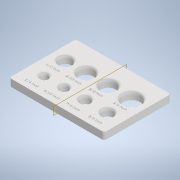
# Autodesk Inventor part: inchHexSocketSetOf8
Saved by Autodesk Inventor 2020.3 (Build 243373000, 373)
## iProperties
Created: 2020-03-13
Part Number: inchHexSocketSetOf8
Material: Generic
Document SubType Name: Modeling
Designer: robst
Density: 1 g/cm^3
Appearance: Default
Author: robst
Autodesk Inventor part; units mm, degrees
(part 1 of 2)
ref_plane "XZ Plane" through (0, 0, 0) normal (0, 1, 0) x (-1, 0, 0)
ref_plane "XY Plane" through (0, 0, 0) normal (0, 0, 1) x (1, 0, 0)
sketch "Sketch1" plane through (0, 0, 0) normal (0, 1, 0) x (-1, 0, 0)
  line L0 (63.5, 44.45) -> (-63.5, 44.45)
  line L1 (-63.5, 44.45) -> (-63.5, -44.45)
  line L2 (-63.5, -44.45) -> (63.5, -44.45)
  line L3 (63.5, -44.45) -> (63.5, 44.45)
  line L4 (63.5, 44.45) -> (-63.5, -44.45) construction
  line L5 (-63.5, 44.45) -> (63.5, -44.45) construction
  point P0 (0, 0)
  dimension "d3" = 88.9
  dimension "d13" = 127
  constraints: 12 end point, 2 midpoint, 2 parallel, 1 horizontal, 1 perpendicular
  measures "d3" distance of L2.end L0.start
  measures "d13" distance of L1.end L2.end
extrude "Extrusion1" add sketch "Sketch1" against normal blind 9.525
sketch "Sketch4" plane through (0, 0, 0) normal (0, 1, 0) x (1, 0, 0)
  line L0 (-63.5, -44.45) -> (-63.5, 44.45) construction
  line L1 (-63.5, -19.05) -> (63.5, -19.05) construction
  line L2 (63.5, 44.45) -> (63.5, -44.45) construction
  line L3 (-63.5, -44.45) -> (63.5, -44.45) projected
  circle A0 centre (-42.0827, -19.05) radius 4.699
  circle A1 centre (-15.4584, -19.05) radius 5.207
  circle A2 centre (12.6898, -19.05) radius 6.223
  circle A3 centre (42.7431, -19.05) radius 7.112
  line L4 (-63.5, 12.7) -> (63.5, 12.7) construction
  circle A4 centre (-45.6692, 12.7) radius 8.128
  circle A5 centre (-17.8054, 12.7) radius 10.033
  circle A6 centre (11.8364, 12.7) radius 9.906
  circle A7 centre (43.0657, 12.7) radius 11.6205
  point P0 (0, 0)
  dimension "d16" = 25.4
  dimension "hex1_4inchHole" = 9.398
  dimension "gap0" = 16.7183
  dimension "hex5_16inchHole" = 10.414
  dimension "gap1" = 26.6243
  dimension "hex3_8inchHole" = 12.446
  dimension "gap2" = 28.1483
  dimension "gap3" = 30.0533
  dimension "hex7_16inchHole" = 14.224
  dimension "frontToBackRowGap" = 31.75
  dimension "gap5" = 9.7028
  dimension "hex1_2inchHole" = 16.256
  dimension "hex9_16inchHole" = 20.066
  dimension "gap6" = 27.8638
  dimension "hex5_8inchHole" = 19.812
  dimension "gap7" = 29.6418
  dimension "hex3_4inchHole" = 23.241
  dimension "gap8" = 31.2293
  dimension "d37" = 8.8138
  dimension "d57" = 13.6449
  constraints: 12 point on line, 8 centre point, 4 end point, 1 horizontal, 1 perpendicular
  measures "d16" distance between parallel lines of L1 L3
  measures "hex1_4inchHole" diameter of A0
  measures "gap0" distance edge to line of A0 L0
  measures "hex5_16inchHole" diameter of A1
  measures "gap1" distance of A1.centre A0.centre
  measures "hex3_8inchHole" diameter of A2
  measures "gap2" distance of A2.centre A1.centre
  measures "gap3" distance of A3.centre A2.centre
  measures "hex7_16inchHole" diameter of A3
  measures "frontToBackRowGap" distance between parallel lines of L4 L1
  measures "gap5" distance edge to line of A4 L0
  measures "hex1_2inchHole" diameter of A4
  measures "hex9_16inchHole" diameter of A5
  measures "gap6" distance of A5.centre A4.centre
  measures "hex5_8inchHole" diameter of A6
  measures "gap7" distance of A6.centre A5.centre
  measures "hex3_4inchHole" diameter of A7
  measures "gap8" distance of A7.centre A6.centre
  measures "d37" distance edge to line of A7 L2
  measures "d57" distance edge to line of A3 L2
extrude "Extrusion3" cut sketch "Sketch4" against normal through all
sketch "Sketch7" plane through (0, 0, 0) normal (0, 1, 0) x (1, 0, 0)
  circle A0 centre (-42.0827, -19.05) radius 4.699 construction
  line L0 (63.5, -44.45) -> (-63.5, -44.45) construction
  line L1 (-46.7817, -35.6779) -> (-37.3837, -35.6779) construction
  line L2 (-20.6654, -35.6779) -> (-10.2514, -35.6779) construction
  line L3 (6.4668, -35.6779) -> (18.9128, -35.6779) construction
  line L4 (35.6311, -35.6779) -> (49.8551, -35.6779) construction
  line L5 (-53.7972, -3.81) -> (-37.5412, -3.81) construction
  line L6 (-27.8384, -3.9984) -> (-7.7724, -3.9984) construction
  line L7 (1.9304, -3.8276) -> (21.7424, -3.8276) construction
  line L8 (31.4452, -3.6244) -> (56.0832, -3.6244) construction
  line L9 (-20.6654, -35.6779) -> (-20.6654, -19.05) construction
  circle A1 centre (-15.4584, -19.05) radius 5.207 construction
  line L10 (-10.2514, -35.6779) -> (-10.2514, -19.05) construction
  line L11 (-46.7817, -19.05) -> (-46.7817, -35.6779) construction
  line L12 (-37.3837, -35.6779) -> (-37.3837, -19.05) construction
  line L13 (6.4668, -35.6779) -> (6.4668, -19.05) construction
  circle A2 centre (12.6898, -19.05) radius 6.223 construction
  line L14 (18.9128, -35.6779) -> (18.9128, -19.05) construction
  line L15 (49.8551, -35.6779) -> (49.8551, -19.05) construction
  circle A3 centre (42.7431, -19.05) radius 7.112 construction
  line L16 (35.6311, -35.6779) -> (35.6311, -19.05) construction
  circle A4 centre (-45.6692, 12.7) radius 8.128 construction
  line L17 (-53.7972, 12.7) -> (-53.7972, -3.81) construction
  line L18 (-37.5412, 12.7) -> (-37.5412, -3.81) construction
  circle A5 centre (-17.8054, 12.7) radius 10.033 construction
  line L19 (-27.8384, 12.7) -> (-27.8384, -3.9984) construction
  line L20 (-7.7724, 12.7) -> (-7.7724, -3.9984) construction
  circle A6 centre (11.8364, 12.7) radius 9.906 construction
  line L21 (1.9304, 12.7) -> (1.9304, -3.8276) construction
  line L22 (21.7424, 12.7) -> (21.7424, -3.8276) construction
  circle A7 centre (43.0657, 12.7) radius 11.6205 construction
  line L23 (31.4452, 12.7) -> (31.4452, -3.6244) construction
  line L24 (56.0832, 12.702) -> (56.0832, -3.6244) construction
  line L25 (-52.169, -5.334) -> (-54.1821, -5.334)
  line L26 (-54.1821, -5.334) -> (-54.1821, -4.8029)
  line L27 (-54.1821, -4.8029) -> (-53.5399, -4.8029)
  line L28 (-53.5399, -4.8029) -> (-53.5399, -3.19)
  line L29 (-53.5399, -3.19) -> (-54.1821, -3.19)
  line L30 (-54.1821, -3.19) -> (-54.1821, -2.6936)
  spline S0 degree 2 poles (-54.1821, -2.6936) (-54.0413, -2.6936) (-53.7622, -2.6565) (-53.6782, -2.617) knots 0 0 0 1 2 2 2
  spline S1 degree 2 poles (-53.6782, -2.617) (-53.5819, -2.5676) (-53.4732, -2.4021) (-53.4633, -2.2786) knots 0 0 0 1 2 2 2
  line L31 (-53.4633, -2.2786) -> (-52.7964, -2.2786)
  line L32 (-52.7964, -2.2786) -> (-52.7964, -4.8029)
  line L33 (-52.7964, -4.8029) -> (-52.169, -4.8029)
  line L34 (-52.169, -4.8029) -> (-52.169, -5.334)
  line L35 (-49.8695, -2.1501) -> (-51.0822, -5.996)
  line L36 (-51.0822, -5.996) -> (-51.6701, -5.996)
  line L37 (-51.6701, -5.996) -> (-50.4598, -2.1501)
  line L38 (-50.4598, -2.1501) -> (-49.8695, -2.1501)
  line L39 (-46.945, -5.334) -> (-49.1853, -5.334)
  line L40 (-49.1853, -5.334) -> (-49.1853, -4.8375)
  spline S2 degree 2 poles (-49.1853, -4.8375) (-48.9012, -4.6103) (-48.4467, -4.2101) (-48.2763, -4.0298) knots 0 0 0 1 2 2 2
  spline S3 degree 2 poles (-48.2763, -4.0298) (-48.0515, -3.7952) (-47.8515, -3.437) (-47.8515, -3.2493) knots 0 0 0 1 2 2 2
  spline S4 degree 2 poles (-47.8515, -3.2493) (-47.8515, -3.0369) (-48.1059, -2.8096) (-48.3331, -2.8096) knots 0 0 0 1 2 2 2
  spline S5 degree 2 poles (-48.3331, -2.8096) (-48.4492, -2.8096) (-48.6567, -2.8665) (-48.7629, -2.9109) knots 0 0 0 1 2 2 2
  spline S6 degree 2 poles (-48.7629, -2.9109) (-48.8666, -2.9578) (-49.0148, -3.0566) (-49.0519, -3.0813) knots 0 0 0 1 2 2 2
  line L41 (-49.0519, -3.0813) -> (-49.1112, -3.0813)
  line L42 (-49.1112, -3.0813) -> (-49.1112, -2.4169)
  spline S7 degree 2 poles (-49.1112, -2.4169) (-48.9827, -2.3552) (-48.4344, -2.2267) (-48.18, -2.2267) knots 0 0 0 1 2 2 2
  spline S8 degree 2 poles (-48.18, -2.2267) (-47.6366, -2.2267) (-47.0783, -2.7108) (-47.0783, -3.148) knots 0 0 0 1 2 2 2
  spline S9 degree 2 poles (-47.0783, -3.148) (-47.0783, -3.4173) (-47.3328, -3.936) (-47.6267, -4.2324) knots 0 0 0 1 2 2 2
  spline S10 degree 2 poles (-47.6267, -4.2324) (-47.8119, -4.4152) (-48.1602, -4.6992) (-48.2368, -4.7585) knots 0 0 0 1 2 2 2
  line L43 (-48.2368, -4.7585) -> (-46.945, -4.7585)
  line L44 (-46.945, -4.7585) -> (-46.945, -5.334)
  line L45 (-44.6059, -5.334) -> (-45.3222, -5.334)
  line L46 (-45.3222, -5.334) -> (-45.3222, -3.0344)
  line L47 (-45.3222, -3.0344) -> (-44.6059, -3.0344)
  line L48 (-44.6059, -3.0344) -> (-44.6059, -5.334)
  line L49 (-44.5836, -2.7059) -> (-45.3419, -2.7059)
  line L50 (-45.3419, -2.7059) -> (-45.3419, -2.1477)
  line L51 (-45.3419, -2.1477) -> (-44.5836, -2.1477)
  line L52 (-44.5836, -2.1477) -> (-44.5836, -2.7059)
  line L53 (-41.9061, -5.334) -> (-42.6274, -5.334)
  line L54 (-42.6274, -5.334) -> (-42.6274, -4.1953)
  spline S11 degree 2 poles (-42.6274, -4.1953) (-42.6274, -4.0545) (-42.6496, -3.7779) (-42.6792, -3.7137) knots 0 0 0 1 2 2 2
  spline S12 degree 2 poles (-42.6792, -3.7137) (-42.7163, -3.6346) (-42.8546, -3.5679) (-42.9732, -3.5679) knots 0 0 0 1 2 2 2
  spline S13 degree 2 poles (-42.9732, -3.5679) (-43.0596, -3.5679) (-43.2399, -3.6346) (-43.3412, -3.7063) knots 0 0 0 1 2 2 2
  line L55 (-43.3412, -3.7063) -> (-43.3412, -5.334)
  line L56 (-43.3412, -5.334) -> (-44.0575, -5.334)
  line L57 (-44.0575, -5.334) -> (-44.0575, -3.0344)
  line L58 (-44.0575, -3.0344) -> (-43.3412, -3.0344)
  line L59 (-43.3412, -3.0344) -> (-43.3412, -3.2888)
  spline S14 degree 2 poles (-43.3412, -3.2888) (-43.1658, -3.1406) (-42.8324, -2.9727) (-42.6298, -2.9727) knots 0 0 0 1 2 2 2
  spline S15 degree 2 poles (-42.6298, -2.9727) (-42.2791, -2.9727) (-41.9061, -3.4173) (-41.9061, -3.8372) knots 0 0 0 1 2 2 2
  line L60 (-41.9061, -3.8372) -> (-41.9061, -5.334)
  spline S16 degree 2 poles (-40.2487, -5.3958) (-40.5328, -5.3958) (-41.0046, -5.2525) (-41.1799, -5.1043) knots 0 0 0 1 2 2 2
  spline S17 degree 2 poles (-41.1799, -5.1043) (-41.3504, -4.9536) (-41.543, -4.5016) (-41.543, -4.1953) knots 0 0 0 1 2 2 2
  spline S18 degree 2 poles (-41.543, -4.1953) (-41.543, -3.8643) (-41.3356, -3.4024) (-41.1552, -3.2542) knots 0 0 0 1 2 2 2
  spline S19 degree 2 poles (-41.1552, -3.2542) (-40.9848, -3.111) (-40.5205, -2.9727) (-40.2685, -2.9727) knots 0 0 0 1 2 2 2
  spline S20 degree 2 poles (-40.2685, -2.9727) (-40.0783, -2.9727) (-39.6979, -3.0616) (-39.5053, -3.1579) knots 0 0 0 1 2 2 2
  line L61 (-39.5053, -3.1579) -> (-39.5053, -3.7705)
  line L62 (-39.5053, -3.7705) -> (-39.5967, -3.7705)
  spline S21 degree 2 poles (-39.5967, -3.7705) (-39.6411, -3.7285) (-39.7646, -3.6297) (-39.8387, -3.5902) knots 0 0 0 1 2 2 2
  spline S22 degree 2 poles (-39.8387, -3.5902) (-39.9178, -3.5457) (-40.1129, -3.4864) (-40.2339, -3.4864) knots 0 0 0 1 2 2 2
  spline S23 degree 2 poles (-40.2339, -3.4864) (-40.5081, -3.4864) (-40.8094, -3.8693) (-40.8094, -4.1953) knots 0 0 0 1 2 2 2
  spline S24 degree 2 poles (-40.8094, -4.1953) (-40.8094, -4.5411) (-40.4883, -4.882) (-40.2216, -4.882) knots 0 0 0 1 2 2 2
  spline S25 degree 2 poles (-40.2216, -4.882) (-40.0857, -4.882) (-39.8832, -4.8202) (-39.8091, -4.7758) knots 0 0 0 1 2 2 2
  spline S26 degree 2 poles (-39.8091, -4.7758) (-39.7375, -4.7338) (-39.6337, -4.6399) (-39.5967, -4.6029) knots 0 0 0 1 2 2 2
  line L63 (-39.5967, -4.6029) -> (-39.5053, -4.6029)
  line L64 (-39.5053, -4.6029) -> (-39.5053, -5.2179)
  spline S27 degree 2 poles (-39.5053, -5.2179) (-39.567, -5.2451) (-39.7276, -5.3142) (-39.8116, -5.3365) knots 0 0 0 1 2 2 2
  spline S28 degree 2 poles (-39.8116, -5.3365) (-39.9153, -5.3661) (-40.0981, -5.3958) (-40.2487, -5.3958) knots 0 0 0 1 2 2 2
  line L65 (-37.013, -5.334) -> (-37.7343, -5.334)
  line L66 (-37.7343, -5.334) -> (-37.7343, -4.1953)
  spline S29 degree 2 poles (-37.7343, -4.1953) (-37.7343, -4.0545) (-37.7565, -3.7779) (-37.7861, -3.7137) knots 0 0 0 1 2 2 2
  spline S30 degree 2 poles (-37.7861, -3.7137) (-37.8232, -3.6346) (-37.9615, -3.5679) (-38.0801, -3.5679) knots 0 0 0 1 2 2 2
  spline S31 degree 2 poles (-38.0801, -3.5679) (-38.1665, -3.5679) (-38.3468, -3.6346) (-38.4481, -3.7063) knots 0 0 0 1 2 2 2
  line L67 (-38.4481, -3.7063) -> (-38.4481, -5.334)
  line L68 (-38.4481, -5.334) -> (-39.1644, -5.334)
  line L69 (-39.1644, -5.334) -> (-39.1644, -2.1501)
  line L70 (-39.1644, -2.1501) -> (-38.4481, -2.1501)
  line L71 (-38.4481, -2.1501) -> (-38.4481, -3.2888)
  spline S32 degree 2 poles (-38.4481, -3.2888) (-38.2727, -3.1406) (-37.9393, -2.9727) (-37.7367, -2.9727) knots 0 0 0 1 2 2 2
  spline S33 degree 2 poles (-37.7367, -2.9727) (-37.386, -2.9727) (-37.013, -3.4173) (-37.013, -3.8372) knots 0 0 0 1 2 2 2
  line L72 (-37.013, -3.8372) -> (-37.013, -5.334)
  spline S34 degree 2 poles (-25.5835, -3.828) (-25.5835, -4.2158) (-25.7638, -4.863) (-25.954, -5.0951) knots 0 0 0 1 2 2 2
  spline S35 degree 2 poles (-25.954, -5.0951) (-26.1516, -5.3298) (-26.7345, -5.5817) (-27.1594, -5.5817) knots 0 0 0 1 2 2 2
  spline S36 degree 2 poles (-27.1594, -5.5817) (-27.3026, -5.5817) (-27.6138, -5.5447) (-27.6657, -5.5299) knots 0 0 0 1 2 2 2
  line L73 (-27.6657, -5.5299) -> (-27.6657, -4.9321)
  line L74 (-27.6657, -4.9321) -> (-27.6064, -4.9321)
  spline S37 degree 2 poles (-27.6064, -4.9321) (-27.5496, -4.9618) (-27.3372, -5.026) (-27.1519, -5.026) knots 0 0 0 1 2 2 2
  spline S38 degree 2 poles (-27.1519, -5.026) (-27.0013, -5.026) (-26.7222, -4.9469) (-26.6234, -4.8605) knots 0 0 0 1 2 2 2
  spline S39 degree 2 poles (-26.6234, -4.8605) (-26.5171, -4.7691) (-26.3788, -4.4999) (-26.3541, -4.2973) knots 0 0 0 1 2 2 2
  spline S40 degree 2 poles (-26.3541, -4.2973) (-26.5171, -4.3986) (-26.7987, -4.5073) (-27.0087, -4.5073) knots 0 0 0 1 2 2 2
  spline S41 degree 2 poles (-27.0087, -4.5073) (-27.1643, -4.5073) (-27.4533, -4.4233) (-27.5718, -4.3344) knots 0 0 0 1 2 2 2
  spline S42 degree 2 poles (-27.5718, -4.3344) (-27.7299, -4.2133) (-27.9152, -3.8255) (-27.9152, -3.5193) knots 0 0 0 1 2 2 2
  spline S43 degree 2 poles (-27.9152, -3.5193) (-27.9152, -3.2797) (-27.7522, -2.8771) (-27.604, -2.7289) knots 0 0 0 1 2 2 2
  spline S44 degree 2 poles (-27.604, -2.7289) (-27.4558, -2.5807) (-27.026, -2.4127) (-26.7617, -2.4127) knots 0 0 0 1 2 2 2
  spline S45 degree 2 poles (-26.7617, -2.4127) (-26.4949, -2.4127) (-26.0824, -2.5609) (-25.9342, -2.7165) knots 0 0 0 1 2 2 2
  spline S46 degree 2 poles (-25.9342, -2.7165) (-25.7613, -2.8894) (-25.5835, -3.4378) (-25.5835, -3.828) knots 0 0 0 1 2 2 2
  spline S47 degree 2 poles (-26.3418, -3.7144) (-26.3418, -3.4649) (-26.4258, -3.1438) (-26.5023, -3.0549) knots 0 0 0 1 2 2 2
  spline S48 degree 2 poles (-26.5023, -3.0549) (-26.5542, -2.9882) (-26.6876, -2.9314) (-26.7641, -2.9314) knots 0 0 0 1 2 2 2
  spline S49 degree 2 poles (-26.7641, -2.9314) (-26.8333, -2.9314) (-26.9618, -2.9857) (-27.021, -3.0549) knots 0 0 0 1 2 2 2
  spline S50 degree 2 poles (-27.021, -3.0549) (-27.0729, -3.1142) (-27.147, -3.3439) (-27.147, -3.4797) knots 0 0 0 1 2 2 2
  spline S51 degree 2 poles (-27.147, -3.4797) (-27.147, -3.6279) (-27.0704, -3.8181) (-27.0062, -3.8749) knots 0 0 0 1 2 2 2
  spline S52 degree 2 poles (-27.0062, -3.8749) (-26.9395, -3.9318) (-26.774, -3.9762) (-26.6703, -3.9762) knots 0 0 0 1 2 2 2
  spline S53 degree 2 poles (-26.6703, -3.9762) (-26.5838, -3.9762) (-26.4035, -3.9293) (-26.3467, -3.9046) knots 0 0 0 1 2 2 2
  spline S54 degree 2 poles (-26.3467, -3.9046) (-26.3467, -3.8824) (-26.3418, -3.7984) (-26.3418, -3.7144) knots 0 0 0 1 2 2 2
  line L75 (-23.3407, -2.3386) -> (-24.5535, -6.1844)
  line L76 (-24.5535, -6.1844) -> (-25.1413, -6.1844)
  line L77 (-25.1413, -6.1844) -> (-23.931, -2.3386)
  line L78 (-23.931, -2.3386) -> (-23.3407, -2.3386)
  line L79 (-20.5521, -5.5224) -> (-22.5651, -5.5224)
  line L80 (-22.5651, -5.5224) -> (-22.5651, -4.9914)
  line L81 (-22.5651, -4.9914) -> (-21.9229, -4.9914)
  line L82 (-21.9229, -4.9914) -> (-21.9229, -3.3785)
  line L83 (-21.9229, -3.3785) -> (-22.5651, -3.3785)
  line L84 (-22.5651, -3.3785) -> (-22.5651, -2.882)
  spline S55 degree 2 poles (-22.5651, -2.882) (-22.4243, -2.882) (-22.1452, -2.8449) (-22.0612, -2.8054) knots 0 0 0 1 2 2 2
  spline S56 degree 2 poles (-22.0612, -2.8054) (-21.9649, -2.756) (-21.8562, -2.5905) (-21.8463, -2.467) knots 0 0 0 1 2 2 2
  line L85 (-21.8463, -2.467) -> (-21.1794, -2.467)
  line L86 (-21.1794, -2.467) -> (-21.1794, -4.9914)
  line L87 (-21.1794, -4.9914) -> (-20.5521, -4.9914)
  line L88 (-20.5521, -4.9914) -> (-20.5521, -5.5224)
  spline S57 degree 2 poles (-17.7634, -4.485) (-17.7634, -4.9667) (-18.3735, -5.5867) (-18.907, -5.5867) knots 0 0 0 1 2 2 2
  spline S58 degree 2 poles (-18.907, -5.5867) (-19.1738, -5.5867) (-19.5912, -5.4335) (-19.737, -5.2829) knots 0 0 0 1 2 2 2
  spline S59 degree 2 poles (-19.737, -5.2829) (-19.9099, -5.1075) (-20.0951, -4.5517) (-20.0951, -4.1639) knots 0 0 0 1 2 2 2
  spline S60 degree 2 poles (-20.0951, -4.1639) (-20.0951, -3.7638) (-19.9222, -3.1414) (-19.7271, -2.9018) knots 0 0 0 1 2 2 2
  spline S61 degree 2 poles (-19.7271, -2.9018) (-19.5418, -2.6745) (-18.9391, -2.4176) (-18.5266, -2.4176) knots 0 0 0 1 2 2 2
  spline S62 degree 2 poles (-18.5266, -2.4176) (-18.376, -2.4176) (-18.0746, -2.4572) (-18.0203, -2.4695) knots 0 0 0 1 2 2 2
  line L89 (-18.0203, -2.4695) -> (-18.0203, -3.0673)
  line L90 (-18.0203, -3.0673) -> (-18.0746, -3.0673)
  spline S63 degree 2 poles (-18.0746, -3.0673) (-18.129, -3.0401) (-18.376, -2.9734) (-18.5341, -2.9734) knots 0 0 0 1 2 2 2
  spline S64 degree 2 poles (-18.5341, -2.9734) (-18.8922, -2.9734) (-19.2825, -3.3513) (-19.3294, -3.702) knots 0 0 0 1 2 2 2
  spline S65 degree 2 poles (-19.3294, -3.702) (-19.1787, -3.6057) (-18.87, -3.4921) (-18.6748, -3.4921) knots 0 0 0 1 2 2 2
  spline S66 degree 2 poles (-18.6748, -3.4921) (-18.5094, -3.4921) (-18.2204, -3.581) (-18.1092, -3.665) knots 0 0 0 1 2 2 2
  spline S67 degree 2 poles (-18.1092, -3.665) (-17.9511, -3.786) (-17.7634, -4.1788) (-17.7634, -4.485) knots 0 0 0 1 2 2 2
  spline S68 degree 2 poles (-18.6551, -4.9445) (-18.5958, -4.8704) (-18.5316, -4.6975) (-18.5316, -4.5221) knots 0 0 0 1 2 2 2
  spline S69 degree 2 poles (-18.5316, -4.5221) (-18.5316, -4.3739) (-18.6057, -4.1812) (-18.6724, -4.1244) knots 0 0 0 1 2 2 2
  spline S70 degree 2 poles (-18.6724, -4.1244) (-18.7415, -4.0651) (-18.912, -4.0231) (-19.0083, -4.0231) knots 0 0 0 1 2 2 2
  spline S71 degree 2 poles (-19.0083, -4.0231) (-19.0898, -4.0231) (-19.2578, -4.0651) (-19.3319, -4.0948) knots 0 0 0 1 2 2 2
  spline S72 degree 2 poles (-19.3319, -4.0948) (-19.3319, -4.1145) (-19.3368, -4.2084) (-19.3368, -4.28) knots 0 0 0 1 2 2 2
  spline S73 degree 2 poles (-19.3368, -4.28) (-19.3368, -4.5443) (-19.2454, -4.863) (-19.1738, -4.9445) knots 0 0 0 1 2 2 2
  spline S74 degree 2 poles (-19.1738, -4.9445) (-19.1219, -5.0112) (-18.9836, -5.068) (-18.9095, -5.068) knots 0 0 0 1 2 2 2
  spline S75 degree 2 poles (-18.9095, -5.068) (-18.8477, -5.068) (-18.7045, -5.0062) (-18.6551, -4.9445) knots 0 0 0 1 2 2 2
  line L91 (-15.407, -5.5224) -> (-16.1233, -5.5224)
  line L92 (-16.1233, -5.5224) -> (-16.1233, -3.2229)
  line L93 (-16.1233, -3.2229) -> (-15.407, -3.2229)
  line L94 (-15.407, -3.2229) -> (-15.407, -5.5224)
  line L95 (-15.3848, -2.8944) -> (-16.1431, -2.8944)
  line L96 (-16.1431, -2.8944) -> (-16.1431, -2.3361)
  line L97 (-16.1431, -2.3361) -> (-15.3848, -2.3361)
  line L98 (-15.3848, -2.3361) -> (-15.3848, -2.8944)
  line L99 (-12.7073, -5.5224) -> (-13.4285, -5.5224)
  line L100 (-13.4285, -5.5224) -> (-13.4285, -4.3838)
  spline S76 degree 2 poles (-13.4285, -4.3838) (-13.4285, -4.243) (-13.4508, -3.9663) (-13.4804, -3.9021) knots 0 0 0 1 2 2 2
  spline S77 degree 2 poles (-13.4804, -3.9021) (-13.5175, -3.8231) (-13.6558, -3.7564) (-13.7743, -3.7564) knots 0 0 0 1 2 2 2
  spline S78 degree 2 poles (-13.7743, -3.7564) (-13.8608, -3.7564) (-14.0411, -3.8231) (-14.1424, -3.8947) knots 0 0 0 1 2 2 2
  line L101 (-14.1424, -3.8947) -> (-14.1424, -5.5224)
  line L102 (-14.1424, -5.5224) -> (-14.8587, -5.5224)
  line L103 (-14.8587, -5.5224) -> (-14.8587, -3.2229)
  line L104 (-14.8587, -3.2229) -> (-14.1424, -3.2229)
  line L105 (-14.1424, -3.2229) -> (-14.1424, -3.4773)
  spline S79 degree 2 poles (-14.1424, -3.4773) (-13.967, -3.3291) (-13.6335, -3.1611) (-13.431, -3.1611) knots 0 0 0 1 2 2 2
  spline S80 degree 2 poles (-13.431, -3.1611) (-13.0803, -3.1611) (-12.7073, -3.6057) (-12.7073, -4.0256) knots 0 0 0 1 2 2 2
  line L106 (-12.7073, -4.0256) -> (-12.7073, -5.5224)
  spline S81 degree 2 poles (-11.0499, -5.5842) (-11.334, -5.5842) (-11.8057, -5.4409) (-11.9811, -5.2927) knots 0 0 0 1 2 2 2
  spline S82 degree 2 poles (-11.9811, -5.2927) (-12.1515, -5.1421) (-12.3442, -4.6901) (-12.3442, -4.3838) knots 0 0 0 1 2 2 2
  spline S83 degree 2 poles (-12.3442, -4.3838) (-12.3442, -4.0528) (-12.1367, -3.5909) (-11.9564, -3.4427) knots 0 0 0 1 2 2 2
  spline S84 degree 2 poles (-11.9564, -3.4427) (-11.786, -3.2994) (-11.3216, -3.1611) (-11.0697, -3.1611) knots 0 0 0 1 2 2 2
  spline S85 degree 2 poles (-11.0697, -3.1611) (-10.8795, -3.1611) (-10.4991, -3.25) (-10.3064, -3.3464) knots 0 0 0 1 2 2 2
  line L107 (-10.3064, -3.3464) -> (-10.3064, -3.9589)
  line L108 (-10.3064, -3.9589) -> (-10.3978, -3.9589)
  spline S86 degree 2 poles (-10.3978, -3.9589) (-10.4423, -3.9169) (-10.5658, -3.8181) (-10.6399, -3.7786) knots 0 0 0 1 2 2 2
  spline S87 degree 2 poles (-10.6399, -3.7786) (-10.7189, -3.7342) (-10.9141, -3.6749) (-11.0351, -3.6749) knots 0 0 0 1 2 2 2
  spline S88 degree 2 poles (-11.0351, -3.6749) (-11.3093, -3.6749) (-11.6106, -4.0577) (-11.6106, -4.3838) knots 0 0 0 1 2 2 2
  spline S89 degree 2 poles (-11.6106, -4.3838) (-11.6106, -4.7296) (-11.2895, -5.0704) (-11.0227, -5.0704) knots 0 0 0 1 2 2 2
  spline S90 degree 2 poles (-11.0227, -5.0704) (-10.8869, -5.0704) (-10.6843, -5.0087) (-10.6102, -4.9642) knots 0 0 0 1 2 2 2
  spline S91 degree 2 poles (-10.6102, -4.9642) (-10.5386, -4.9222) (-10.4349, -4.8284) (-10.3978, -4.7913) knots 0 0 0 1 2 2 2
  line L109 (-10.3978, -4.7913) -> (-10.3064, -4.7913)
  line L110 (-10.3064, -4.7913) -> (-10.3064, -5.4064)
  spline S92 degree 2 poles (-10.3064, -5.4064) (-10.3682, -5.4335) (-10.5287, -5.5027) (-10.6127, -5.5249) knots 0 0 0 1 2 2 2
  spline S93 degree 2 poles (-10.6127, -5.5249) (-10.7165, -5.5546) (-10.8992, -5.5842) (-11.0499, -5.5842) knots 0 0 0 1 2 2 2
  line L111 (-7.8142, -5.5224) -> (-8.5354, -5.5224)
  line L112 (-8.5354, -5.5224) -> (-8.5354, -4.3838)
  spline S94 degree 2 poles (-8.5354, -4.3838) (-8.5354, -4.243) (-8.5577, -3.9663) (-8.5873, -3.9021) knots 0 0 0 1 2 2 2
  spline S95 degree 2 poles (-8.5873, -3.9021) (-8.6243, -3.8231) (-8.7627, -3.7564) (-8.8812, -3.7564) knots 0 0 0 1 2 2 2
  spline S96 degree 2 poles (-8.8812, -3.7564) (-8.9677, -3.7564) (-9.148, -3.8231) (-9.2493, -3.8947) knots 0 0 0 1 2 2 2
  line L113 (-9.2493, -3.8947) -> (-9.2493, -5.5224)
  line L114 (-9.2493, -5.5224) -> (-9.9656, -5.5224)
  line L115 (-9.9656, -5.5224) -> (-9.9656, -2.3386)
  line L116 (-9.9656, -2.3386) -> (-9.2493, -2.3386)
  line L117 (-9.2493, -2.3386) -> (-9.2493, -3.4773)
  spline S97 degree 2 poles (-9.2493, -3.4773) (-9.0739, -3.3291) (-8.7404, -3.1611) (-8.5379, -3.1611) knots 0 0 0 1 2 2 2
  spline S98 degree 2 poles (-8.5379, -3.1611) (-8.1872, -3.1611) (-7.8142, -3.6057) (-7.8142, -4.0256) knots 0 0 0 1 2 2 2
  line L118 (-7.8142, -4.0256) -> (-7.8142, -5.5224)
  spline S99 degree 2 poles (5.4032, -4.3191) (5.4032, -4.5587) (5.2402, -4.9638) (5.0797, -5.1095) knots 0 0 0 1 2 2 2
  spline S100 degree 2 poles (5.0797, -5.1095) (4.9191, -5.2552) (4.4795, -5.4158) (4.1584, -5.4158) knots 0 0 0 1 2 2 2
  spline S101 degree 2 poles (4.1584, -5.4158) (3.8175, -5.4133) (3.3284, -5.3022) (3.1679, -5.2305) knots 0 0 0 1 2 2 2
  line L119 (3.1679, -5.2305) -> (3.1679, -4.5661)
  line L120 (3.1679, -4.5661) -> (3.237, -4.5661)
  spline S102 degree 2 poles (3.237, -4.5661) (3.2963, -4.5982) (3.4396, -4.6822) (3.5557, -4.7267) knots 0 0 0 1 2 2 2
  spline S103 degree 2 poles (3.5557, -4.7267) (3.6644, -4.7687) (3.8891, -4.8255) (4.025, -4.8255) knots 0 0 0 1 2 2 2
  spline S104 degree 2 poles (4.025, -4.8255) (4.1435, -4.8255) (4.4202, -4.7662) (4.5042, -4.6871) knots 0 0 0 1 2 2 2
  spline S105 degree 2 poles (4.5042, -4.6871) (4.5659, -4.6254) (4.6351, -4.4747) (4.6351, -4.3487) knots 0 0 0 1 2 2 2
  spline S106 degree 2 poles (4.6351, -4.3487) (4.6351, -4.2401) (4.5461, -4.0869) (4.4745, -4.04) knots 0 0 0 1 2 2 2
  spline S107 degree 2 poles (4.4745, -4.04) (4.3708, -3.9708) (4.0744, -3.9313) (3.9682, -3.9313) knots 0 0 0 1 2 2 2
  spline S108 degree 2 poles (3.9682, -3.9313) (3.8002, -3.9313) (3.4816, -3.9857) (3.3655, -4.0153) knots 0 0 0 1 2 2 2
  line L121 (3.3655, -4.0153) -> (3.2988, -4.0153)
  line L122 (3.2988, -4.0153) -> (3.2988, -2.3036)
  line L123 (3.2988, -2.3036) -> (5.3193, -2.3036)
  line L124 (5.3193, -2.3036) -> (5.3193, -2.8791)
  line L125 (5.3193, -2.8791) -> (4.0225, -2.8791)
  line L126 (4.0225, -2.8791) -> (4.0225, -3.3854)
  spline S109 degree 2 poles (4.0225, -3.3854) (4.0843, -3.3805) (4.2547, -3.3756) (4.3016, -3.3756) knots 0 0 0 1 2 2 2
  spline S110 degree 2 poles (4.3016, -3.3756) (4.5214, -3.3756) (4.8919, -3.4645) (5.0377, -3.5559) knots 0 0 0 1 2 2 2
  spline S111 degree 2 poles (5.0377, -3.5559) (5.2106, -3.6695) (5.4032, -4.0474) (5.4032, -4.3191) knots 0 0 0 1 2 2 2
  line L127 (7.6361, -2.1677) -> (6.4234, -6.0135)
  line L128 (6.4234, -6.0135) -> (5.8355, -6.0135)
  line L129 (5.8355, -6.0135) -> (7.0458, -2.1677)
  line L130 (7.0458, -2.1677) -> (7.6361, -2.1677)
  spline S112 degree 2 poles (10.5532, -4.5044) (10.5532, -4.6995) (10.3902, -5.0379) (10.2346, -5.1614) knots 0 0 0 1 2 2 2
  spline S113 degree 2 poles (10.2346, -5.1614) (10.079, -5.2849) (9.6319, -5.4232) (9.3429, -5.4232) knots 0 0 0 1 2 2 2
  spline S114 degree 2 poles (9.3429, -5.4232) (9.0342, -5.4232) (8.5723, -5.2824) (8.4241, -5.1614) knots 0 0 0 1 2 2 2
  spline S115 degree 2 poles (8.4241, -5.1614) (8.2783, -5.0404) (8.14, -4.7118) (8.14, -4.5291) knots 0 0 0 1 2 2 2
  spline S116 degree 2 poles (8.14, -4.5291) (8.14, -4.2672) (8.429, -3.919) (8.7032, -3.8029) knots 0 0 0 1 2 2 2
  line L131 (8.7032, -3.8029) -> (8.7032, -3.7905)
  spline S117 degree 2 poles (8.7032, -3.7905) (8.434, -3.6596) (8.2215, -3.2866) (8.2215, -3.0569) knots 0 0 0 1 2 2 2
  spline S118 degree 2 poles (8.2215, -3.0569) (8.2215, -2.889) (8.3697, -2.595) (8.5155, -2.4789) knots 0 0 0 1 2 2 2
  spline S119 degree 2 poles (8.5155, -2.4789) (8.6563, -2.3678) (9.0836, -2.2344) (9.3503, -2.2344) knots 0 0 0 1 2 2 2
  spline S120 degree 2 poles (9.3503, -2.2344) (9.6319, -2.2344) (10.0518, -2.3554) (10.1877, -2.4542) knots 0 0 0 1 2 2 2
  spline S121 degree 2 poles (10.1877, -2.4542) (10.326, -2.553) (10.4742, -2.8396) (10.4742, -3.0051) knots 0 0 0 1 2 2 2
  spline S122 degree 2 poles (10.4742, -3.0051) (10.4742, -3.2224) (10.2222, -3.5707) (9.9629, -3.6917) knots 0 0 0 1 2 2 2
  line L132 (9.9629, -3.6917) -> (9.9629, -3.7016)
  spline S123 degree 2 poles (9.9629, -3.7016) (10.2667, -3.8251) (10.5532, -4.2252) (10.5532, -4.5044) knots 0 0 0 1 2 2 2
  spline S124 degree 2 poles (9.7974, -4.5365) (9.7974, -4.3858) (9.669, -4.2277) (9.4615, -4.1264) knots 0 0 0 1 2 2 2
  spline S125 degree 2 poles (9.4615, -4.1264) (9.4022, -4.0993) (9.1774, -4.0128) (9.091, -3.9758) knots 0 0 0 1 2 2 2
  spline S126 degree 2 poles (9.091, -3.9758) (9.0119, -4.0548) (8.886, -4.2919) (8.886, -4.4327) knots 0 0 0 1 2 2 2
  spline S127 degree 2 poles (8.886, -4.4327) (8.886, -4.6452) (9.1577, -4.8996) (9.3775, -4.8996) knots 0 0 0 1 2 2 2
  spline S128 degree 2 poles (9.3775, -4.8996) (9.4392, -4.8996) (9.5924, -4.86) (9.6517, -4.8205) knots 0 0 0 1 2 2 2
  spline S129 degree 2 poles (9.6517, -4.8205) (9.7184, -4.7736) (9.7974, -4.6452) (9.7974, -4.5365) knots 0 0 0 1 2 2 2
  spline S130 degree 2 poles (9.7307, -3.094) (9.7307, -2.9384) (9.5257, -2.7531) (9.3503, -2.7531) knots 0 0 0 1 2 2 2
  spline S131 degree 2 poles (9.3503, -2.7531) (9.1824, -2.7531) (8.9774, -2.9211) (8.9774, -3.0446) knots 0 0 0 1 2 2 2
  spline S132 degree 2 poles (8.9774, -3.0446) (8.9774, -3.1656) (9.1009, -3.3163) (9.2318, -3.378) knots 0 0 0 1 2 2 2
  spline S133 degree 2 poles (9.2318, -3.378) (9.2886, -3.4077) (9.4467, -3.4694) (9.5776, -3.5188) knots 0 0 0 1 2 2 2
  spline S134 degree 2 poles (9.5776, -3.5188) (9.6566, -3.4151) (9.7307, -3.22) (9.7307, -3.094) knots 0 0 0 1 2 2 2
  line L133 (12.8997, -5.3516) -> (12.1834, -5.3516)
  line L134 (12.1834, -5.3516) -> (12.1834, -3.052)
  line L135 (12.1834, -3.052) -> (12.8997, -3.052)
  line L136 (12.8997, -3.052) -> (12.8997, -5.3516)
  line L137 (12.922, -2.7235) -> (12.1637, -2.7235)
  line L138 (12.1637, -2.7235) -> (12.1637, -2.1653)
  line L139 (12.1637, -2.1653) -> (12.922, -2.1653)
  line L140 (12.922, -2.1653) -> (12.922, -2.7235)
  line L141 (15.5995, -5.3516) -> (14.8782, -5.3516)
  line L142 (14.8782, -5.3516) -> (14.8782, -4.2129)
  spline S135 degree 2 poles (14.8782, -4.2129) (14.8782, -4.0721) (14.856, -3.7955) (14.8264, -3.7312) knots 0 0 0 1 2 2 2
  spline S136 degree 2 poles (14.8264, -3.7312) (14.7893, -3.6522) (14.651, -3.5855) (14.5324, -3.5855) knots 0 0 0 1 2 2 2
  spline S137 degree 2 poles (14.5324, -3.5855) (14.446, -3.5855) (14.2657, -3.6522) (14.1644, -3.7238) knots 0 0 0 1 2 2 2
  line L143 (14.1644, -3.7238) -> (14.1644, -5.3516)
  line L144 (14.1644, -5.3516) -> (13.4481, -5.3516)
  line L145 (13.4481, -5.3516) -> (13.4481, -3.052)
  line L146 (13.4481, -3.052) -> (14.1644, -3.052)
  line L147 (14.1644, -3.052) -> (14.1644, -3.3064)
  spline S138 degree 2 poles (14.1644, -3.3064) (14.3398, -3.1582) (14.6732, -2.9902) (14.8758, -2.9902) knots 0 0 0 1 2 2 2
  spline S139 degree 2 poles (14.8758, -2.9902) (15.2265, -2.9902) (15.5995, -3.4348) (15.5995, -3.8547) knots 0 0 0 1 2 2 2
  line L148 (15.5995, -3.8547) -> (15.5995, -5.3516)
  spline S140 degree 2 poles (17.2569, -5.4133) (16.9728, -5.4133) (16.501, -5.2701) (16.3257, -5.1219) knots 0 0 0 1 2 2 2
  spline S141 degree 2 poles (16.3257, -5.1219) (16.1552, -4.9712) (15.9626, -4.5192) (15.9626, -4.2129) knots 0 0 0 1 2 2 2
  spline S142 degree 2 poles (15.9626, -4.2129) (15.9626, -3.8819) (16.17, -3.42) (16.3504, -3.2718) knots 0 0 0 1 2 2 2
  spline S143 degree 2 poles (16.3504, -3.2718) (16.5208, -3.1286) (16.9851, -2.9902) (17.2371, -2.9902) knots 0 0 0 1 2 2 2
  spline S144 degree 2 poles (17.2371, -2.9902) (17.4273, -2.9902) (17.8077, -3.0792) (18.0003, -3.1755) knots 0 0 0 1 2 2 2
  line L149 (18.0003, -3.1755) -> (18.0003, -3.7881)
  line L150 (18.0003, -3.7881) -> (17.9089, -3.7881)
  spline S145 degree 2 poles (17.9089, -3.7881) (17.8645, -3.7461) (17.741, -3.6473) (17.6669, -3.6077) knots 0 0 0 1 2 2 2
  spline S146 degree 2 poles (17.6669, -3.6077) (17.5878, -3.5633) (17.3927, -3.504) (17.2717, -3.504) knots 0 0 0 1 2 2 2
  spline S147 degree 2 poles (17.2717, -3.504) (16.9975, -3.504) (16.6962, -3.8869) (16.6962, -4.2129) knots 0 0 0 1 2 2 2
  spline S148 degree 2 poles (16.6962, -4.2129) (16.6962, -4.5587) (17.0173, -4.8996) (17.284, -4.8996) knots 0 0 0 1 2 2 2
  spline S149 degree 2 poles (17.284, -4.8996) (17.4199, -4.8996) (17.6224, -4.8378) (17.6965, -4.7934) knots 0 0 0 1 2 2 2
  spline S150 degree 2 poles (17.6965, -4.7934) (17.7681, -4.7514) (17.8719, -4.6575) (17.9089, -4.6205) knots 0 0 0 1 2 2 2
  line L151 (17.9089, -4.6205) -> (18.0003, -4.6205)
  line L152 (18.0003, -4.6205) -> (18.0003, -5.2355)
  spline S151 degree 2 poles (18.0003, -5.2355) (17.9386, -5.2627) (17.778, -5.3318) (17.694, -5.354) knots 0 0 0 1 2 2 2
  spline S152 degree 2 poles (17.694, -5.354) (17.5903, -5.3837) (17.4075, -5.4133) (17.2569, -5.4133) knots 0 0 0 1 2 2 2
  line L153 (20.4926, -5.3516) -> (19.7713, -5.3516)
  line L154 (19.7713, -5.3516) -> (19.7713, -4.2129)
  spline S153 degree 2 poles (19.7713, -4.2129) (19.7713, -4.0721) (19.7491, -3.7955) (19.7195, -3.7312) knots 0 0 0 1 2 2 2
  spline S154 degree 2 poles (19.7195, -3.7312) (19.6824, -3.6522) (19.5441, -3.5855) (19.4255, -3.5855) knots 0 0 0 1 2 2 2
  spline S155 degree 2 poles (19.4255, -3.5855) (19.3391, -3.5855) (19.1588, -3.6522) (19.0575, -3.7238) knots 0 0 0 1 2 2 2
  line L155 (19.0575, -3.7238) -> (19.0575, -5.3516)
  line L156 (19.0575, -5.3516) -> (18.3412, -5.3516)
  line L157 (18.3412, -5.3516) -> (18.3412, -2.1677)
  line L158 (18.3412, -2.1677) -> (19.0575, -2.1677)
  line L159 (19.0575, -2.1677) -> (19.0575, -3.3064)
  spline S156 degree 2 poles (19.0575, -3.3064) (19.2329, -3.1582) (19.5663, -2.9902) (19.7689, -2.9902) knots 0 0 0 1 2 2 2
  spline S157 degree 2 poles (19.7689, -2.9902) (20.1196, -2.9902) (20.4926, -3.4348) (20.4926, -3.8547) knots 0 0 0 1 2 2 2
  line L160 (20.4926, -3.8547) -> (20.4926, -5.3516)
  spline S158 degree 2 poles (37.3236, -4.2246) (37.3236, -4.4494) (37.1581, -4.8174) (36.9976, -4.9459) knots 0 0 0 1 2 2 2
  spline S159 degree 2 poles (36.9976, -4.9459) (36.837, -5.0743) (36.3998, -5.2126) (36.0862, -5.2126) knots 0 0 0 1 2 2 2
  spline S160 degree 2 poles (36.0862, -5.2126) (35.7305, -5.2126) (35.2216, -5.0941) (35.0611, -5.02) knots 0 0 0 1 2 2 2
  line L161 (35.0611, -5.02) -> (35.0611, -4.358)
  line L162 (35.0611, -4.358) -> (35.1352, -4.358)
  spline S161 degree 2 poles (35.1352, -4.358) (35.3032, -4.4642) (35.7552, -4.6223) (35.9429, -4.6223) knots 0 0 0 1 2 2 2
  spline S162 degree 2 poles (35.9429, -4.6223) (36.054, -4.6223) (36.3134, -4.5828) (36.4023, -4.5186) knots 0 0 0 1 2 2 2
  spline S163 degree 2 poles (36.4023, -4.5186) (36.4715, -4.4667) (36.5555, -4.316) (36.5555, -4.1802) knots 0 0 0 1 2 2 2
  spline S164 degree 2 poles (36.5555, -4.1802) (36.5555, -4.0443) (36.4369, -3.8986) (36.3381, -3.864) knots 0 0 0 1 2 2 2
  spline S165 degree 2 poles (36.3381, -3.864) (36.2393, -3.8294) (35.9651, -3.822) (35.8589, -3.822) knots 0 0 0 1 2 2 2
  line L163 (35.8589, -3.822) -> (35.728, -3.822)
  line L164 (35.728, -3.822) -> (35.728, -3.286)
  line L165 (35.728, -3.286) -> (35.849, -3.286)
  spline S166 degree 2 poles (35.849, -3.286) (35.9874, -3.286) (36.222, -3.2613) (36.3035, -3.2243) knots 0 0 0 1 2 2 2
  spline S167 degree 2 poles (36.3035, -3.2243) (36.385, -3.1847) (36.4764, -3.0464) (36.4764, -2.9279) knots 0 0 0 1 2 2 2
  spline S168 degree 2 poles (36.4764, -2.9279) (36.4764, -2.834) (36.39, -2.7179) (36.3282, -2.6858) knots 0 0 0 1 2 2 2
  spline S169 degree 2 poles (36.3282, -2.6858) (36.2541, -2.6488) (36.0565, -2.6241) (35.9874, -2.6241) knots 0 0 0 1 2 2 2
  spline S170 degree 2 poles (35.9874, -2.6241) (35.8762, -2.6241) (35.6416, -2.6759) (35.5329, -2.7179) knots 0 0 0 1 2 2 2
  spline S171 degree 2 poles (35.5329, -2.7179) (35.4464, -2.75) (35.2587, -2.8538) (35.2142, -2.8809) knots 0 0 0 1 2 2 2
  line L166 (35.2142, -2.8809) -> (35.15, -2.8809)
  line L167 (35.15, -2.8809) -> (35.15, -2.2288)
  spline S172 degree 2 poles (35.15, -2.2288) (35.3081, -2.1622) (35.8416, -2.0362) (36.1207, -2.0362) knots 0 0 0 1 2 2 2
  spline S173 degree 2 poles (36.1207, -2.0362) (36.3924, -2.0362) (36.7926, -2.13) (36.9334, -2.2214) knots 0 0 0 1 2 2 2
  spline S174 degree 2 poles (36.9334, -2.2214) (37.089, -2.3178) (37.2446, -2.6142) (37.2446, -2.7994) knots 0 0 0 1 2 2 2
  spline S175 degree 2 poles (37.2446, -2.7994) (37.2446, -3.0612) (36.9433, -3.4515) (36.6962, -3.5083) knots 0 0 0 1 2 2 2
  line L168 (36.6962, -3.5083) -> (36.6962, -3.538)
  spline S176 degree 2 poles (36.6962, -3.538) (36.8049, -3.5528) (37.0124, -3.6318) (37.1112, -3.7207) knots 0 0 0 1 2 2 2
  spline S177 degree 2 poles (37.1112, -3.7207) (37.2026, -3.7998) (37.3236, -4.0517) (37.3236, -4.2246) knots 0 0 0 1 2 2 2
  line L169 (39.5639, -1.9646) -> (38.3512, -5.8104)
  line L170 (38.3512, -5.8104) -> (37.7633, -5.8104)
  line L171 (37.7633, -5.8104) -> (38.9736, -1.9646)
  line L172 (38.9736, -1.9646) -> (39.5639, -1.9646)
  line L173 (42.5255, -4.437) -> (42.113, -4.437)
  line L174 (42.113, -4.437) -> (42.113, -5.1558)
  line L175 (42.113, -5.1558) -> (41.3745, -5.1558)
  line L176 (41.3745, -5.1558) -> (41.3745, -4.437)
  line L177 (41.3745, -4.437) -> (40.0308, -4.437)
  line L178 (40.0308, -4.437) -> (40.0308, -3.8689)
  line L179 (40.0308, -3.8689) -> (41.3498, -2.1004)
  line L180 (41.3498, -2.1004) -> (42.113, -2.1004)
  line L181 (42.113, -2.1004) -> (42.113, -3.8887)
  line L182 (42.113, -3.8887) -> (42.5255, -3.8887)
  line L183 (42.5255, -3.8887) -> (42.5255, -4.437)
  line L184 (41.3745, -3.8887) -> (41.3745, -2.8513)
  line L185 (41.3745, -2.8513) -> (40.6013, -3.8887)
  line L186 (40.6013, -3.8887) -> (41.3745, -3.8887)
  line L187 (44.8275, -5.1484) -> (44.1112, -5.1484)
  line L188 (44.1112, -5.1484) -> (44.1112, -2.8488)
  line L189 (44.1112, -2.8488) -> (44.8275, -2.8488)
  line L190 (44.8275, -2.8488) -> (44.8275, -5.1484)
  line L191 (44.8498, -2.5203) -> (44.0915, -2.5203)
  line L192 (44.0915, -2.5203) -> (44.0915, -1.9621)
  line L193 (44.0915, -1.9621) -> (44.8498, -1.9621)
  line L194 (44.8498, -1.9621) -> (44.8498, -2.5203)
  line L195 (47.5273, -5.1484) -> (46.806, -5.1484)
  line L196 (46.806, -5.1484) -> (46.806, -4.0097)
  spline S178 degree 2 poles (46.806, -4.0097) (46.806, -3.8689) (46.7838, -3.5923) (46.7542, -3.5281) knots 0 0 0 1 2 2 2
  spline S179 degree 2 poles (46.7542, -3.5281) (46.7171, -3.449) (46.5788, -3.3823) (46.4602, -3.3823) knots 0 0 0 1 2 2 2
  spline S180 degree 2 poles (46.4602, -3.3823) (46.3738, -3.3823) (46.1935, -3.449) (46.0922, -3.5207) knots 0 0 0 1 2 2 2
  line L197 (46.0922, -3.5207) -> (46.0922, -5.1484)
  line L198 (46.0922, -5.1484) -> (45.3759, -5.1484)
  line L199 (45.3759, -5.1484) -> (45.3759, -2.8488)
  line L200 (45.3759, -2.8488) -> (46.0922, -2.8488)
  line L201 (46.0922, -2.8488) -> (46.0922, -3.1032)
  spline S181 degree 2 poles (46.0922, -3.1032) (46.2676, -2.955) (46.601, -2.7871) (46.8036, -2.7871) knots 0 0 0 1 2 2 2
  spline S182 degree 2 poles (46.8036, -2.7871) (47.1543, -2.7871) (47.5273, -3.2317) (47.5273, -3.6516) knots 0 0 0 1 2 2 2
  line L202 (47.5273, -3.6516) -> (47.5273, -5.1484)
  spline S183 degree 2 poles (49.1847, -5.2102) (48.9006, -5.2102) (48.4288, -5.0669) (48.2535, -4.9187) knots 0 0 0 1 2 2 2
  spline S184 degree 2 poles (48.2535, -4.9187) (48.083, -4.768) (47.8904, -4.316) (47.8904, -4.0097) knots 0 0 0 1 2 2 2
  spline S185 degree 2 poles (47.8904, -4.0097) (47.8904, -3.6787) (48.0978, -3.2169) (48.2782, -3.0687) knots 0 0 0 1 2 2 2
  spline S186 degree 2 poles (48.2782, -3.0687) (48.4486, -2.9254) (48.9129, -2.7871) (49.1649, -2.7871) knots 0 0 0 1 2 2 2
  spline S187 degree 2 poles (49.1649, -2.7871) (49.3551, -2.7871) (49.7355, -2.876) (49.9281, -2.9723) knots 0 0 0 1 2 2 2
  line L203 (49.9281, -2.9723) -> (49.9281, -3.5849)
  line L204 (49.9281, -3.5849) -> (49.8367, -3.5849)
  spline S188 degree 2 poles (49.8367, -3.5849) (49.7923, -3.5429) (49.6688, -3.4441) (49.5947, -3.4046) knots 0 0 0 1 2 2 2
  spline S189 degree 2 poles (49.5947, -3.4046) (49.5156, -3.3601) (49.3205, -3.3008) (49.1995, -3.3008) knots 0 0 0 1 2 2 2
  spline S190 degree 2 poles (49.1995, -3.3008) (48.9253, -3.3008) (48.624, -3.6837) (48.624, -4.0097) knots 0 0 0 1 2 2 2
  spline S191 degree 2 poles (48.624, -4.0097) (48.624, -4.3555) (48.9451, -4.6964) (49.2118, -4.6964) knots 0 0 0 1 2 2 2
  spline S192 degree 2 poles (49.2118, -4.6964) (49.3477, -4.6964) (49.5502, -4.6346) (49.6243, -4.5902) knots 0 0 0 1 2 2 2
  spline S193 degree 2 poles (49.6243, -4.5902) (49.6959, -4.5482) (49.7997, -4.4543) (49.8367, -4.4173) knots 0 0 0 1 2 2 2
  line L205 (49.8367, -4.4173) -> (49.9281, -4.4173)
  line L206 (49.9281, -4.4173) -> (49.9281, -5.0323)
  spline S194 degree 2 poles (49.9281, -5.0323) (49.8664, -5.0595) (49.7058, -5.1286) (49.6218, -5.1509) knots 0 0 0 1 2 2 2
  spline S195 degree 2 poles (49.6218, -5.1509) (49.5181, -5.1805) (49.3353, -5.2102) (49.1847, -5.2102) knots 0 0 0 1 2 2 2
  line L207 (52.4204, -5.1484) -> (51.6991, -5.1484)
  line L208 (51.6991, -5.1484) -> (51.6991, -4.0097)
  spline S196 degree 2 poles (51.6991, -4.0097) (51.6991, -3.8689) (51.6769, -3.5923) (51.6473, -3.5281) knots 0 0 0 1 2 2 2
  spline S197 degree 2 poles (51.6473, -3.5281) (51.6102, -3.449) (51.4719, -3.3823) (51.3533, -3.3823) knots 0 0 0 1 2 2 2
  spline S198 degree 2 poles (51.3533, -3.3823) (51.2669, -3.3823) (51.0866, -3.449) (50.9853, -3.5207) knots 0 0 0 1 2 2 2
  line L209 (50.9853, -3.5207) -> (50.9853, -5.1484)
  line L210 (50.9853, -5.1484) -> (50.269, -5.1484)
  line L211 (50.269, -5.1484) -> (50.269, -1.9646)
  line L212 (50.269, -1.9646) -> (50.9853, -1.9646)
  line L213 (50.9853, -1.9646) -> (50.9853, -3.1032)
  spline S199 degree 2 poles (50.9853, -3.1032) (51.1607, -2.955) (51.4941, -2.7871) (51.6967, -2.7871) knots 0 0 0 1 2 2 2
  spline S200 degree 2 poles (51.6967, -2.7871) (52.0474, -2.7871) (52.4204, -3.2317) (52.4204, -3.6516) knots 0 0 0 1 2 2 2
  line L214 (52.4204, -3.6516) -> (52.4204, -5.1484)
  line L215 (-48.5826, -37.2019) -> (-50.5956, -37.2019)
  line L216 (-50.5956, -37.2019) -> (-50.5956, -36.6708)
  line L217 (-50.5956, -36.6708) -> (-49.9534, -36.6708)
  line L218 (-49.9534, -36.6708) -> (-49.9534, -35.0579)
  line L219 (-49.9534, -35.0579) -> (-50.5956, -35.0579)
  line L220 (-50.5956, -35.0579) -> (-50.5956, -34.5614)
  spline S201 degree 2 poles (-50.5956, -34.5614) (-50.4548, -34.5614) (-50.1757, -34.5244) (-50.0917, -34.4848) knots 0 0 0 1 2 2 2
  spline S202 degree 2 poles (-50.0917, -34.4848) (-49.9954, -34.4354) (-49.8867, -34.27) (-49.8769, -34.1465) knots 0 0 0 1 2 2 2
  line L221 (-49.8769, -34.1465) -> (-49.21, -34.1465)
  line L222 (-49.21, -34.1465) -> (-49.21, -36.6708)
  line L223 (-49.21, -36.6708) -> (-48.5826, -36.6708)
  line L224 (-48.5826, -36.6708) -> (-48.5826, -37.2019)
  line L225 (-46.283, -34.018) -> (-47.4958, -37.8638)
  line L226 (-47.4958, -37.8638) -> (-48.0836, -37.8638)
  line L227 (-48.0836, -37.8638) -> (-46.8733, -34.018)
  line L228 (-46.8733, -34.018) -> (-46.283, -34.018)
  line L229 (-43.3214, -36.4905) -> (-43.7339, -36.4905)
  line L230 (-43.7339, -36.4905) -> (-43.7339, -37.2093)
  line L231 (-43.7339, -37.2093) -> (-44.4725, -37.2093)
  line L232 (-44.4725, -37.2093) -> (-44.4725, -36.4905)
  line L233 (-44.4725, -36.4905) -> (-45.8161, -36.4905)
  line L234 (-45.8161, -36.4905) -> (-45.8161, -35.9224)
  line L235 (-45.8161, -35.9224) -> (-44.4972, -34.1539)
  line L236 (-44.4972, -34.1539) -> (-43.7339, -34.1539)
  line L237 (-43.7339, -34.1539) -> (-43.7339, -35.9422)
  line L238 (-43.7339, -35.9422) -> (-43.3214, -35.9422)
  line L239 (-43.3214, -35.9422) -> (-43.3214, -36.4905)
  line L240 (-44.4725, -35.9422) -> (-44.4725, -34.9048)
  line L241 (-44.4725, -34.9048) -> (-45.2456, -35.9422)
  line L242 (-45.2456, -35.9422) -> (-44.4725, -35.9422)
  line L243 (-41.0194, -37.2019) -> (-41.7357, -37.2019)
  line L244 (-41.7357, -37.2019) -> (-41.7357, -34.9023)
  line L245 (-41.7357, -34.9023) -> (-41.0194, -34.9023)
  line L246 (-41.0194, -34.9023) -> (-41.0194, -37.2019)
  line L247 (-40.9971, -34.5738) -> (-41.7554, -34.5738)
  line L248 (-41.7554, -34.5738) -> (-41.7554, -34.0155)
  line L249 (-41.7554, -34.0155) -> (-40.9971, -34.0155)
  line L250 (-40.9971, -34.0155) -> (-40.9971, -34.5738)
  line L251 (-38.3197, -37.2019) -> (-39.0409, -37.2019)
  line L252 (-39.0409, -37.2019) -> (-39.0409, -36.0632)
  spline S203 degree 2 poles (-39.0409, -36.0632) (-39.0409, -35.9224) (-39.0631, -35.6458) (-39.0928, -35.5815) knots 0 0 0 1 2 2 2
  spline S204 degree 2 poles (-39.0928, -35.5815) (-39.1298, -35.5025) (-39.2681, -35.4358) (-39.3867, -35.4358) knots 0 0 0 1 2 2 2
  spline S205 degree 2 poles (-39.3867, -35.4358) (-39.4731, -35.4358) (-39.6535, -35.5025) (-39.7547, -35.5741) knots 0 0 0 1 2 2 2
  line L253 (-39.7547, -35.5741) -> (-39.7547, -37.2019)
  line L254 (-39.7547, -37.2019) -> (-40.471, -37.2019)
  line L255 (-40.471, -37.2019) -> (-40.471, -34.9023)
  line L256 (-40.471, -34.9023) -> (-39.7547, -34.9023)
  line L257 (-39.7547, -34.9023) -> (-39.7547, -35.1567)
  spline S206 degree 2 poles (-39.7547, -35.1567) (-39.5794, -35.0085) (-39.2459, -34.8405) (-39.0434, -34.8405) knots 0 0 0 1 2 2 2
  spline S207 degree 2 poles (-39.0434, -34.8405) (-38.6926, -34.8405) (-38.3197, -35.2851) (-38.3197, -35.705) knots 0 0 0 1 2 2 2
  line L258 (-38.3197, -35.705) -> (-38.3197, -37.2019)
  spline S208 degree 2 poles (-36.6623, -37.2636) (-36.9463, -37.2636) (-37.4181, -37.1204) (-37.5935, -36.9722) knots 0 0 0 1 2 2 2
  spline S209 degree 2 poles (-37.5935, -36.9722) (-37.7639, -36.8215) (-37.9566, -36.3695) (-37.9566, -36.0632) knots 0 0 0 1 2 2 2
  spline S210 degree 2 poles (-37.9566, -36.0632) (-37.9566, -35.7322) (-37.7491, -35.2703) (-37.5688, -35.1221) knots 0 0 0 1 2 2 2
  spline S211 degree 2 poles (-37.5688, -35.1221) (-37.3983, -34.9789) (-36.934, -34.8405) (-36.682, -34.8405) knots 0 0 0 1 2 2 2
  spline S212 degree 2 poles (-36.682, -34.8405) (-36.4918, -34.8405) (-36.1115, -34.9295) (-35.9188, -35.0258) knots 0 0 0 1 2 2 2
  line L259 (-35.9188, -35.0258) -> (-35.9188, -35.6383)
  line L260 (-35.9188, -35.6383) -> (-36.0102, -35.6383)
  spline S213 degree 2 poles (-36.0102, -35.6383) (-36.0546, -35.5964) (-36.1781, -35.4976) (-36.2522, -35.458) knots 0 0 0 1 2 2 2
  spline S214 degree 2 poles (-36.2522, -35.458) (-36.3313, -35.4136) (-36.5264, -35.3543) (-36.6474, -35.3543) knots 0 0 0 1 2 2 2
  spline S215 degree 2 poles (-36.6474, -35.3543) (-36.9216, -35.3543) (-37.223, -35.7371) (-37.223, -36.0632) knots 0 0 0 1 2 2 2
  spline S216 degree 2 poles (-37.223, -36.0632) (-37.223, -36.409) (-36.9019, -36.7499) (-36.6351, -36.7499) knots 0 0 0 1 2 2 2
  spline S217 degree 2 poles (-36.6351, -36.7499) (-36.4992, -36.7499) (-36.2967, -36.6881) (-36.2226, -36.6436) knots 0 0 0 1 2 2 2
  spline S218 degree 2 poles (-36.2226, -36.6436) (-36.151, -36.6017) (-36.0472, -36.5078) (-36.0102, -36.4707) knots 0 0 0 1 2 2 2
  line L261 (-36.0102, -36.4707) -> (-35.9188, -36.4707)
  line L262 (-35.9188, -36.4707) -> (-35.9188, -37.0858)
  spline S219 degree 2 poles (-35.9188, -37.0858) (-35.9805, -37.1129) (-36.1411, -37.1821) (-36.2251, -37.2043) knots 0 0 0 1 2 2 2
  spline S220 degree 2 poles (-36.2251, -37.2043) (-36.3288, -37.234) (-36.5116, -37.2636) (-36.6623, -37.2636) knots 0 0 0 1 2 2 2
  line L263 (-33.4265, -37.2019) -> (-34.1478, -37.2019)
  line L264 (-34.1478, -37.2019) -> (-34.1478, -36.0632)
  spline S221 degree 2 poles (-34.1478, -36.0632) (-34.1478, -35.9224) (-34.17, -35.6458) (-34.1997, -35.5815) knots 0 0 0 1 2 2 2
  spline S222 degree 2 poles (-34.1997, -35.5815) (-34.2367, -35.5025) (-34.375, -35.4358) (-34.4936, -35.4358) knots 0 0 0 1 2 2 2
  spline S223 degree 2 poles (-34.4936, -35.4358) (-34.58, -35.4358) (-34.7604, -35.5025) (-34.8616, -35.5741) knots 0 0 0 1 2 2 2
  line L265 (-34.8616, -35.5741) -> (-34.8616, -37.2019)
  line L266 (-34.8616, -37.2019) -> (-35.5779, -37.2019)
  line L267 (-35.5779, -37.2019) -> (-35.5779, -34.018)
  line L268 (-35.5779, -34.018) -> (-34.8616, -34.018)
  line L269 (-34.8616, -34.018) -> (-34.8616, -35.1567)
  spline S224 degree 2 poles (-34.8616, -35.1567) (-34.6863, -35.0085) (-34.3528, -34.8405) (-34.1503, -34.8405) knots 0 0 0 1 2 2 2
  spline S225 degree 2 poles (-34.1503, -34.8405) (-33.7995, -34.8405) (-33.4265, -35.2851) (-33.4265, -35.705) knots 0 0 0 1 2 2 2
  line L270 (-33.4265, -35.705) -> (-33.4265, -37.2019)
  spline S226 degree 2 poles (-23.2266, -36.1694) (-23.2266, -36.409) (-23.3897, -36.8141) (-23.5502, -36.9598) knots 0 0 0 1 2 2 2
  spline S227 degree 2 poles (-23.5502, -36.9598) (-23.7108, -37.1055) (-24.1504, -37.2661) (-24.4715, -37.2661) knots 0 0 0 1 2 2 2
  spline S228 degree 2 poles (-24.4715, -37.2661) (-24.8124, -37.2636) (-25.3015, -37.1525) (-25.462, -37.0808) knots 0 0 0 1 2 2 2
  line L271 (-25.462, -37.0808) -> (-25.462, -36.4164)
  line L272 (-25.462, -36.4164) -> (-25.3928, -36.4164)
  spline S229 degree 2 poles (-25.3928, -36.4164) (-25.3336, -36.4485) (-25.1903, -36.5325) (-25.0742, -36.577) knots 0 0 0 1 2 2 2
  spline S230 degree 2 poles (-25.0742, -36.577) (-24.9655, -36.6189) (-24.7408, -36.6758) (-24.6049, -36.6758) knots 0 0 0 1 2 2 2
  spline S231 degree 2 poles (-24.6049, -36.6758) (-24.4863, -36.6758) (-24.2097, -36.6165) (-24.1257, -36.5374) knots 0 0 0 1 2 2 2
  spline S232 degree 2 poles (-24.1257, -36.5374) (-24.064, -36.4757) (-23.9948, -36.325) (-23.9948, -36.199) knots 0 0 0 1 2 2 2
  spline S233 degree 2 poles (-23.9948, -36.199) (-23.9948, -36.0904) (-24.0837, -35.9372) (-24.1554, -35.8903) knots 0 0 0 1 2 2 2
  spline S234 degree 2 poles (-24.1554, -35.8903) (-24.2591, -35.8211) (-24.5555, -35.7816) (-24.6617, -35.7816) knots 0 0 0 1 2 2 2
  spline S235 degree 2 poles (-24.6617, -35.7816) (-24.8297, -35.7816) (-25.1483, -35.8359) (-25.2644, -35.8656) knots 0 0 0 1 2 2 2
  line L273 (-25.2644, -35.8656) -> (-25.3311, -35.8656)
  line L274 (-25.3311, -35.8656) -> (-25.3311, -34.1539)
  line L275 (-25.3311, -34.1539) -> (-23.3106, -34.1539)
  line L276 (-23.3106, -34.1539) -> (-23.3106, -34.7294)
  line L277 (-23.3106, -34.7294) -> (-24.6074, -34.7294)
  line L278 (-24.6074, -34.7294) -> (-24.6074, -35.2357)
  spline S236 degree 2 poles (-24.6074, -35.2357) (-24.5456, -35.2308) (-24.3752, -35.2259) (-24.3283, -35.2259) knots 0 0 0 1 2 2 2
  spline S237 degree 2 poles (-24.3283, -35.2259) (-24.1084, -35.2259) (-23.7379, -35.3148) (-23.5922, -35.4062) knots 0 0 0 1 2 2 2
  spline S238 degree 2 poles (-23.5922, -35.4062) (-23.4193, -35.5198) (-23.2266, -35.8977) (-23.2266, -36.1694) knots 0 0 0 1 2 2 2
  line L279 (-20.9937, -34.018) -> (-22.2065, -37.8638)
  line L280 (-22.2065, -37.8638) -> (-22.7944, -37.8638)
  line L281 (-22.7944, -37.8638) -> (-21.5841, -34.018)
  line L282 (-21.5841, -34.018) -> (-20.9937, -34.018)
  line L283 (-18.2051, -37.2019) -> (-20.2182, -37.2019)